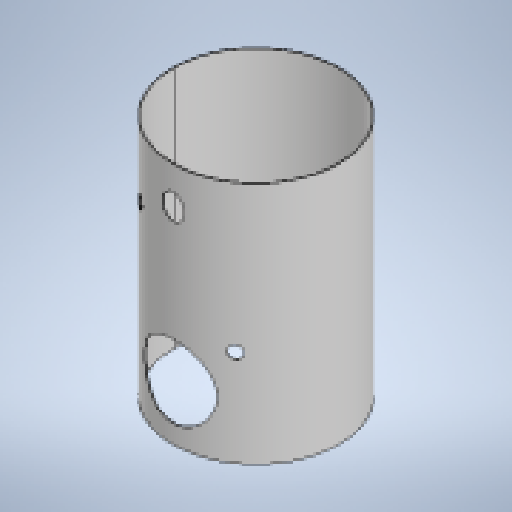
# Autodesk Inventor part: PNS-701 main shell D1200
Saved by Autodesk Inventor 2025.1 (Build 291241020, 241B)
## iProperties
Created: 2025-02-11
Part Number: PNS-701 main shell D1200
Material: Steel
Document SubType Name: Sheet Metal
Designer: pokla
Density: 7.85 g/cm^3
Flat Pattern Width: 180.342 cm
Flat Pattern Length: 378.545 cm
Flat Pattern Area: 68267.6 cm^2
Sheet Metal Rule: Default_mm
Sheet Metal Width: 1803.422 mm
Sheet Metal Length: 3785.447 mm
Sheet Metal Area: 6826756.915 mm^2
Appearance: Default
Mass: 309189 g
Surface Area: 132135 cm^2
Volume: 39387.1 cm^3
Flat Pattern Width: 177 cm
Flat Pattern Area: 67002.4 cm^2
Sheet Metal Width: 1770.000 mm
Sheet Metal Area: 6700241.169 mm^2
Author: pokla
Autodesk Inventor part; units mm, degrees
sketch "Sketch1" plane through (0, 0, 0) normal (0, 1, 0) x (-1, 0, 0)
  line L0 (606, 1803.4216) -> (600, 1803.4216)
  line L1 (600, 1803.4216) -> (600, 0)
  line L2 (600, 0) -> (606, 0)
  line L3 (606, 0) -> (606, 1803.4216)
  line L4 (0, 0) -> (0, 1673.0415)
  point P0 (603, 0)
  dimension "d0" = 6
  dimension "d1" = 1803.4216
  dimension "d2" = 1200
  constraints: 10 end point, 2 parallel, 1 coincident, 1 horizontal, 1 horizontal alignment, 1 midpoint, 1 perpendicular, 1 vertical
  measures "d0" distance between parallel lines of L1 L3
  measures "d1" distance of L2.end L0.start
  measures "d2" diameter of L1 L4
revolve "Revolution1" add sketch "Sketch1" angle 359.9 about axis through (0, 0, 0) along (0, 0, 1)
sketch "Sketch2" plane through (0, 0, 0) normal (0, 1, 0) x (-1, 0, 0)
  circle A0 centre (0, 400) radius 265
  line L0 (600, 1803.4216) -> (-600, 1803.4216) projected
  line L1 (110, 1603.4216) -> (-110, 1603.4216) construction
  line L2 (110, 1693.4216) -> (-110, 1693.4216)
  line L3 (-110, 1513.4216) -> (110, 1513.4216)
  arc A1 (110, 1513.4216) -> (110, 1693.4216) centre (110, 1603.4216) ccw
  arc A2 (-110, 1693.4216) -> (-110, 1513.4216) centre (-110, 1603.4216) ccw
  line L4 (200, 1603.4216) -> (-200, 1603.4216) construction
  point P0 (0, 0)
  point P1 (599.9991, 1803.4216)
  point P2 (0, 1603.4216)
  dimension "d4" = 530
  dimension "d12" = 400
  dimension "d15" = 200
  dimension "d16" = 400
  dimension "d17" = 180
  constraints: 10 end point, 6 point on circle, 4 tangent, 3 centre point, 2 vertical alignment, 1 horizontal, 1 midpoint, 1 parallel
  measures "d4" diameter of A0
  measures "d12" distance of A0.centre point (0, 0)
  measures "d15" distance between parallel lines of L1 L0
  measures "d16" distance of L4.start L4.end
  measures "d17" distance between parallel lines of L3 L2
extrude "Extrusion1" cut sketch "Sketch2" against normal through all contours A0
sketch "floor angle sketch" plane through (0, 0, 0) normal (0, 0, 1) x (1, 0, 0)
  line L0 (0, 0) -> (0, -267.717)
  line L1 (0, -267.717) -> (0, 0)
  line L2 (0, 0) -> (72.6903, -155.8849)
  line L3 (0, 0) -> (-51.6219, -73.7237)
  line L4 (0, 0) -> (51.6219, -73.7237)
  dimension "Feeder_way_angle" = 335
  dimension "Feeder_way_line" = 172
  dimension "Outer_way_line" = 90
  dimension "Inner_way_line" = 90
  dimension "Outer_way_angle" = 325
  dimension "Inner_way_angle" = 35
  constraints: 10 end point, 1 collinear, 1 vertical
  measures "Feeder_way_line" distance of L0.start L2.end
  measures "Outer_way_line" distance of L0.start L4.end
  measures "Inner_way_line" distance of L0.start L3.end
  measures "Inner_way_angle" angle of L0 L3
ref_plane "Feeder Plane" through (0, 0, -10) normal (0.9063, 0.4226, 0) x (0, 0, 1)
sketch "Feeder horisont hight angle" plane through (0, 0, -10) normal (0.9063, 0.4226, 0) x (0, 0, 1)
  line L0 (1813.4216, -600) -> (1813.4216, 600) construction
  line L1 (10, 0) -> (1813.4216, 0) construction
  line L2 (1160.1257, 0) -> (1510, 606)
  line L3 (10, 606) -> (1813.4216, 606) construction
  line L4 (1510, 606) -> (1510, 0) construction
  point P0 (1813.4216, -253.571)
  point P1 (1813.4216, -254.5197)
  dimension "d34" = 1500
  dimension "d35" = 30
  constraints: 6 end point, 3 point on line, 1 midpoint, 1 perpendicular
  measures "d34" distance of L3.start L2.end
  measures "d35" angle of L2 L4
ref_plane "Feeder Work Plane" through (0, 0, 1150.1257) normal (0.366, -0.7849, 0.5) x (0.9063, 0.4226, 0)
sketch "Sketch8" plane through (0, 0, 1150.1257) normal (0.366, -0.7849, 0.5) x (0.9063, 0.4226, 0)
  circle A0 centre (0, 0) radius 86
  point P0 (0, -996.0381)
  point P1 (0, 0)
  dimension "d36" = 172
  constraints: 1 centre point, 1 coincident, 1 vertical alignment
  measures "d36" diameter of A0
extrude "Feeder Extrusion" cut sketch "Sketch8" along normal through all
ref_plane "Inner Plane" through (0, 0, 0) normal (-0.8192, 0.5736, 0) x (-0.5736, -0.8192, 0)
sketch "Inner horisont hight angle" plane through (0, 0, 0) normal (-0.8192, 0.5736, 0) x (-0.5736, -0.8192, 0)
  line L0 (606, 1803.4216) -> (-606, 1803.4216) construction
  line L1 (606, 0) -> (606, 1803.4216) construction
  line L2 (0, 0) -> (0, 1803.4216) construction
  line L3 (0, 1300) -> (606, 1300) construction
  line L4 (606, 1300) -> (0, 1300)
  point P0 (347.5873, 1803.4216)
  point P1 (346.7204, 1803.4216)
  dimension "d40" = 0
  dimension "d41" = 1300
  constraints: 6 end point, 3 point on line, 1 midpoint, 1 perpendicular
  measures "d40" distance between parallel lines of L4 L3
  measures "d41" distance of L1.start L3.end
ref_plane "Inner Work Plane" through (0, 0, 1300) normal (0.5736, 0.8192, 0) x (-0.8192, 0.5736, 0)
sketch "Sketch10" plane through (0, 0, 1300) normal (0.5736, 0.8192, 0) x (-0.8192, 0.5736, 0)
  circle A0 centre (0, 0) radius 45.5
  point P0 (0, -1300)
  point P1 (0, 0)
  point P2 (0, 0)
  point P3 (0, 0)
  dimension "d42" = 91
  constraints: 1 centre point, 1 coincident
  measures "d42" diameter of A0
extrude "Inner Extrusion" cut sketch "Sketch10" against normal through all
ref_plane "Outer Plane" through (0, 0, 0) normal (-0.8192, -0.5736, 0) x (0.5736, -0.8192, 0)
sketch "Sketch11" plane through (0, 0, 0) normal (-0.8192, -0.5736, 0) x (0.5736, -0.8192, 0)
  line L0 (0, 0) -> (0, 1803.4216)
  line L1 (606, 1803.4216) -> (-606, 1803.4216) projected
  line L2 (0, 700) -> (606, 700)
  line L3 (606, 0) -> (606, 1803.4216) projected
  line L4 (606, 700) -> (0, 700)
  point P0 (-347.5873, 1803.4216)
  point P1 (-348.4532, 1803.4216)
  dimension "d45" = 0
  dimension "d46" = 700
  constraints: 6 end point, 3 point on line, 1 midpoint, 1 perpendicular
  measures "d45" distance between parallel lines of L4 L2
  measures "d46" distance of L3.start L2.end
ref_plane "Work Plane9" through (0, 0, 700) normal (-0.5736, 0.8192, 0) x (-0.8192, -0.5736, 0)
sketch "Sketch12" plane through (0, 0, 700) normal (-0.5736, 0.8192, 0) x (-0.8192, -0.5736, 0)
  circle A0 centre (0, 0) radius 46
  point P0 (0, -700)
  point P1 (0, 0)
  point P2 (0, 0)
  point P3 (0, 0)
  dimension "d47" = 92
  constraints: 1 centre point, 1 coincident
  measures "d47" diameter of A0
extrude "Extrusion6" cut sketch "Sketch12" against normal through all
equation "\"d1\" = MAIN_hight - 2 * Disherd_head_hight"
equation "\"d2\" = MAIN_filter_diam"
equation "\"d4\" = Accsess_hatch_diameter"
equation "\"d16\" = Charging_hatch_width"
equation "\"d17\" = Charging_hatch_hight"
equation "\"d34\" = Feedr_hight"
equation "\"d35\" = Feeder_horisont_hight_angle"
equation "\"BendRadius\" = Thickness"
equation "\"BendReliefWidth\" = Thickness"
equation "\"BendReliefDepth\" = 0.5 * Thickness"
equation "\"CornerReliefSize\" = 4 * Thickness"
equation "\"MinimumRemnant\" = 2 * Thickness"
equation "\"TransitionRadius\" = BendRadius"
equation "\"JacobiRadiusSize\" = BendRadius"
equation "\"GapSize\" = Thickness"
equation "\"Feeder_floor_angle\" = 60deg"
equation "\"Feedr_hight\" = 1500"
equation "\"Feeder_horisont_hight_angle\" = 30deg"
equation "\"MAIN_hight\" = 2310"
equation "\"Disherd_head_hight\" = 253.289193"
equation "\"MAIN_filter_diam\" = 1200"
equation "\"Accsess_hatch_diameter\" = 530"
equation "\"Charging_hatch_width\" = 400"
equation "\"Charging_hatch_hight\" = 180"
equation "\"Thickness\" = 6"
body "Solid1"
